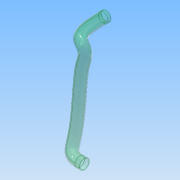
# Autodesk Inventor part: Top_Lower Pipe 5
Saved by Autodesk Inventor 2018.1 (Build 221171000, 171)
## iProperties
Created: 2019-03-21
Part Number: Top_Lower Pipe 5
Material: PMMA Plastic
Document SubType Name: Modeling
Designer: James
Density: 1.188 g/cm^3
Appearance: Clear - Green 1
Author: James
Autodesk Inventor part; units mm, degrees
ref_plane "YZ Plane" through (0, 0, 0) normal (1, 0, 0) x (0, 1, 0)
ref_plane "XZ Plane" through (0, 0, 0) normal (0, 1, 0) x (-1, 0, 0)
ref_plane "XY Plane" through (0, 0, 0) normal (0, 0, 1) x (1, 0, 0)
sketch "Sketch2" plane through (0, 0, 0) normal (0, 1, 0) x (-1, 0, 0)
  circle A0 centre (0, 0) radius 23
  circle A1 centre (0, 0) radius 20
  dimension "d1" = 46
  dimension "d2" = 40
  constraints: 2 centre point, 2 coincident
  measures "d1" diameter of A0
  measures "d2" diameter of A1
sketch3d "3D Sketch1"
  spline S0 degree 4 poles (0, 0, 0) (0, -135, 0) (60, -135, 0) (60, -135, -80) (26, -135, -80) (26, -135, -418) (26, -190, -418) (86, -190, -418) knots 1 1 1 1 1 2 3 4 5 5 5 5 5
  dimension "d24" = 135
  dimension "d25" = 60
  dimension "d26" = 80
  dimension "d27" = 34
  dimension "d28" = 338
  dimension "d29" = 55
  dimension "d30" = 60
sweep "Sweep1" add profiles "Sketch2" path "3D Sketch1"
sketch "Sketch3" plane through (0, 0, 0) normal (0, 1, 0) x (1, 0, 0)
  spline S0 degree 6 poles (-20, 0) (-20, 33.2309) (21.091, 38.0022) (54.9823, 0) (21.091, -38.0022) (-20, -33.2309) (-20, 0) knots 0 0 0 0 0 0 0 1 1 1 1 1 1 1 weights 1.669078 1.03673 1.038347 0.853534 1.038347 1.03673 1.669078 projected
  circle A0 centre (0, 0) radius 23 projected
  point P0 (-23, 0)
  constraints: 1 horizontal alignment, 1 other
extrude "Extrusion1" add sketch "Sketch3" along normal blind 12
sketch "Sketch4" plane through (0, 0, 0) normal (0, 0, 1) x (1, 0, 0)
  line L0 (23, 12) -> (-23, 12) projected
  point P0 (0, 0)
  point P1 (0, 5)
  point P2 (0, 12)
  dimension "d11" = 7
  constraints: 1 midpoint, 1 vertical alignment
  measures "d11" distance from line of L0 point (0, 5)
hole "Hole1" at (0, 5, 0) direction (0, 0, -1) diameter 4.5 end through all
sketch "Sketch5" plane through (86, -190, -418) normal (1, 0, 0) x (0, 0, -1)
  spline S0 degree 6 poles (-3.9754, -19.6009) (28.5924, -26.2062) (41.4362, 13.1164) (10.9289, 53.8852) (-33.0517, 28.2239) (-36.5432, -12.9956) (-3.9754, -19.6009) knots 0 0 0 0 0 0 0 1 1 1 1 1 1 1 weights 1.669078 1.03673 1.038347 0.853534 1.038347 1.03673 1.669078 projected
  circle A0 centre (0, 0) radius 23 projected
  point P0 (-418, 190)
  point P1 (-5.747, -22.2704)
  constraints: 2 other
extrude "Extrusion2" add sketch "Sketch5" along normal blind 20 contours S0 picked at (-21.5933, -3.3898)
body "Solid1"
